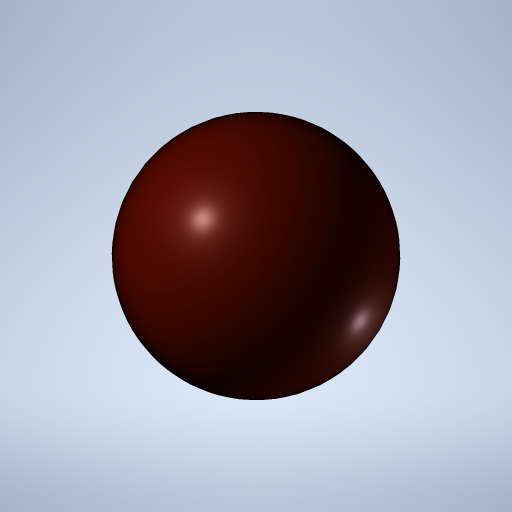
# Autodesk Inventor part: pong_ball
Saved by Autodesk Inventor 2023 (Build 270158000, 158)
## iProperties
Created: 2024-02-11
Part Number: pong_ball
Material: Generic
Document SubType Name: Modeling
Designer: victo
Density: 1 g/cm^3
Appearance: Orange
Author: victo
Autodesk Inventor part; units mm, degrees
ref_plane "YZ Plane" through (0, 0, 0) normal (1, 0, 0) x (0, 1, 0)
ref_plane "XZ Plane" through (0, 0, 0) normal (0, 1, 0) x (-1, 0, 0)
ref_plane "XY Plane" through (0, 0, 0) normal (0, 0, 1) x (1, 0, 0)
sketch "Sketch1" plane through (0, 0, 0) normal (0, 0, 1) x (1, 0, 0)
  arc A0 (0, -15) -> (0, 15) centre (0, 0) ccw
  line L0 (0, 15) -> (0, -15)
  dimension "d0" = 15
  constraints: 2 end point, 2 point on circle, 1 centre point, 1 coincident, 1 vertical
  measures "d0" radius of A0
revolve "Revolution1" add sketch "Sketch1" angle 360 about axis through (0, 15, 0) along (0, -1, 0)
body "Solid1"
